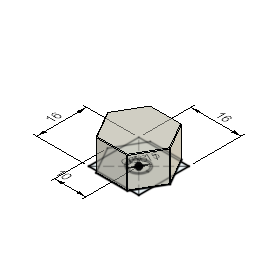
PolyLedCap-v8 (Autodesk Fusion 360 design; units mm, degrees)
Autodesk Fusion 360 part; units mm, degrees
note: some values were not read from the file. Set by a fixed rule: which face or edge a step refers to.
sketch "Sketch1" plane through (0, 0, 0) normal (0, 0, 1) x (1, 0, 0)
  line L0 (8, -8) -> (-8, -8)
  line L1 (-8, -8) -> (-8, 8)
  line L2 (-8, 8) -> (8, 8)
  line L3 (8, 8) -> (8, -8)
  line L4 (8, -8) -> (-8, 8) construction
  line L5 (-8, -8) -> (8, 8) construction
  circle A0 centre (0, 0) radius 2.575
  circle A1 centre (0, 0) radius 3.05
  line L6 (10, 0) -> (5, 8.6603)
  line L7 (5, 8.6603) -> (-5, 8.6603)
  line L8 (-5, 8.6603) -> (-10, 0)
  line L9 (-10, 0) -> (-5, -8.6603)
  line L10 (-5, -8.6603) -> (5, -8.6603)
  line L11 (5, -8.6603) -> (10, 0)
  dimension "d1" = 16
  dimension "d2" = 16
  dimension "d20" = 5.15
  dimension "d23" = 6.1
  dimension "d28" = 10
  constraint horizontal L0
  constraint perpendicular L0 L1
  constraint parallel L0 L2
  constraint parallel L1 L3
  constraint coincident L4 A0.centre
  constraint coincident L5 A0.centre
  constraint coincident A0.centre A1.centre
  constraint horizontal L10
  measures "d1" distance of L1.end L2.end
  measures "d2" distance of L0.end L1.end
  measures "d20" diameter of A0
  measures "d23" diameter of A1
  measures "d28" distance of A0.centre L8.end
extrude "Extrude1" add sketch "Sketch1" along normal blind 10 contours L0 L9 L10 L11 | L0 L1 L2 L3 L6 L8 L9 L11 | L3 L6 L11 | L1 L8 L9 | L2 L6 L7 L8 | A0 | A1
fillet "Fillet1" radius 0.2 15 faces at (-2.6667, -1.1547, 10) (-1.6667, -8.6603, 3.3333) (5.1271, -8.4402, 3.3333) (6.2541, -6.488, 3.3333) (8.6667, -2.3094, 3.3333) (-9.3333, -1.1547, 3.3333) (-7.1271, -4.9761, 6.6667) (-5.2541, -8.2201, 3.3333) (-5.1271, 8.4402, 3.3333) (-6.2541, 6.488, 3.3333) (-8.6667, 2.3094, 3.3333) (1.6667, 8.6603, 3.3333) (9.3333, 1.1547, 3.3333) (7.1271, 4.9761, 3.3333) (5.2541, 8.2201, 3.3333)
extrude "Extrude5" cut sketch "Sketch1" along normal blind 8 contours A0
chamfer "Chamfer3" distance 0.6 angle 45 1 edges at (-2.4007, -0.9312, 0)
